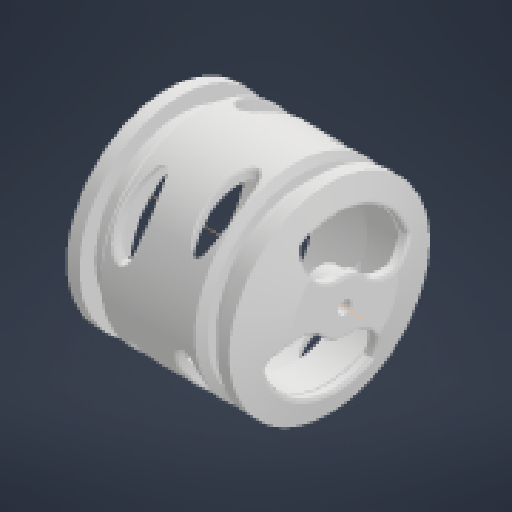
# Autodesk Inventor part: wheel
Saved by Autodesk Inventor 2024 (Build 280153000, 153)
## iProperties
Created: 2023-09-26
Part Number: wheel
Material: Типовые
Document SubType Name: Modeling
Designer: user
Density: 1 g/cm^3
Appearance: По умолчанию
Mass: 47.7551 g
Surface Area: 315.947 cm^2
Volume: 47.7551 cm^3
Author: user
Autodesk Inventor part; units mm, degrees
ref_plane "YZ Plane" through (0, 0, 0) normal (1, 0, 0) x (0, 1, 0)
ref_plane "XZ Plane" through (0, 0, 0) normal (0, 1, 0) x (-1, 0, 0)
sketch "Эскиз1" plane through (0, 0, 0) normal (0, 0, 1) x (1, 0, 0)
  line L0 (0, 0) -> (0, 32)
  line L1 (0, 32) -> (4, 32)
  line L2 (4, 32) -> (4, 27)
  line L3 (4, 27) -> (9, 27)
  line L4 (9, 27) -> (9, 32)
  line L5 (9, 32) -> (43, 32)
  line L6 (43, 32) -> (43, 27)
  line L7 (43, 27) -> (48, 27)
  line L8 (48, 27) -> (48, 32)
  line L9 (48, 32) -> (52, 32)
  line L10 (52, 32) -> (52, 0)
  line L11 (52, 0) -> (0, 0)
  dimension "d0" = 32
  dimension "d1" = 27
  dimension "d2" = 5
  dimension "d3" = 34
  dimension "d4" = 4
  constraints: 24 end point, 8 perpendicular, 6 point on line, 2 collinear, 1 vertical
  measures "d0" distance of L0.start L0.end
  measures "d1" vertical distance of L0.start L2.end
  measures "d2" distance of L2.end L3.end
  measures "d3" distance of L4.end L5.end
  measures "d4" distance of L0.end L1.end
revolve "Вращение1" add sketch "Эскиз1" angle 360 about axis through (52, 0, 0) along (-1, 0, 0)
sketch "Эскиз2" plane through (0, 0, 0) normal (0, 0, 1) x (1, 0, 0)
  line L0 (52, 32) -> (52, -32) projected
  line L1 (52, 32) -> (57, 17)
  line L2 (52, 0) -> (57, 0)
  line L3 (57, 0) -> (57, 17)
  point P0 (0, 0)
  dimension "d6" = 17
  dimension "d7" = 5
  constraints: 6 end point, 1 horizontal, 1 midpoint, 1 perpendicular
  measures "d6" distance of L2.end L1.end
  measures "d7" distance of L2.start L2.end
revolve "Вращение2" add sketch "Эскиз2" angle 360 about axis through (52, 0, 0) along (1, 0, 0)
shell "Оболочка1" thickness 3 removed faces 1 at (0, 9.4449, -4.957)
sketch "Эскиз3" plane through (54, 0, 0) normal (-1, 0, 0) x (0, 0, 1)
  circle A0 centre (0, 0) radius 7.5
  line L0 (-2, -3.4641) -> (-4, 0)
  line L1 (-4, 0) -> (-2, 3.4641)
  line L2 (-2, 3.4641) -> (2, 3.4641)
  line L3 (2, 3.4641) -> (4, 0)
  line L4 (4, 0) -> (2, -3.4641)
  line L5 (2, -3.4641) -> (-2, -3.4641)
  dimension "d10" = 15
  dimension "d11" = 8
  constraints: 12 end point, 2 coincident, 1 centre point, 1 horizontal, 13 other
  measures "d10" diameter of A0
  measures "d11" distance of L0.end L3.end
extrude "Выдавливание1" add sketch "Эскиз3" along normal blind 5.25
sketch "Эскиз4" plane through (54, -3.4641, -2) normal (-1, 0, 0) x (0, 0, 1)
  circle A0 centre (2, 3.4641) radius 7.5 projected
  circle A1 centre (2, 3.4641) radius 2
  dimension "d14" = 4
  constraints: 1 centre point, 1 coincident
  measures "d14" diameter of A1
extrude "Выдавливание2" cut sketch "Эскиз4" against normal through all contours A1
sketch "Эскиз6" plane through (57, 0, 0) normal (1, 0, 0) x (0, 0, -1)
  circle A0 centre (0, 0) radius 24 projected
  arc A1 (5.4637, -6.5114) -> (8.4595, 0.8288) centre (0, 0) ccw
  arc A2 (21.1003, 11.4357) -> (8.4595, 0.8288) centre (18.4118, 1.8039) ccw
  arc A3 (5.4637, -6.5114) -> (7.0727, -22.9342) centre (11.8916, -14.1718) ccw
  line L0 (8.4595, 0.8288) -> (6.271, 23.1662) construction
  line L1 (8.4595, 0.8288) -> (21.1003, 11.4357) construction
  line L2 (5.4637, -6.5114) -> (-11.7297, -20.9383) construction
  line L3 (5.4637, -6.5114) -> (7.0727, -22.9342) construction
  line L4 (0, 0) -> (0, -11.096) construction
  point P0 (0, 0)
  dimension "d26" = 17
  dimension "d29" = 10
  dimension "d31" = 50
  constraints: 10 end point, 10 point on circle, 4 tangent, 3 centre point, 1 coincident, 1 equal radius, 1 parallel, 1 point on line, 1 vertical
  measures "d26" diameter of A1
  measures "d29" radius of A2
  measures "d31" angle of L4 L2
extrude "Выдавливание3" cut sketch "Эскиз6" against normal blind 10 contours A0 A3 A1 A2 picked at (14.0191, -12.4187)
pattern_circular "Круговой массив1" count 2 over 360 about axis through (54.5, 0, 0) along (1, 0, 0) of "Выдавливание3"
ref_plane "РабПлоскость1" through (26, 0, -32) normal (0, 0, 1) x (1, 0, 0)
sketch "Эскиз7" plane through (26, 0, -32) normal (0, 0, 1) x (1, 0, 0)
  ellipse E0 centre (-10, -17) end of major axis (-10, -7) minor radius 4
  ellipse E1 centre (10, 17) end of major axis (10, 7) minor radius 4
  line L0 (-17, 32) -> (-17, -32) construction
  line L1 (17, -32) -> (-17, -32) construction
  line L2 (17, 32) -> (-17, 32) construction
  line L3 (17, 32) -> (17, -32) construction
  point P0 (-26, 0)
  dimension "d41" = 10
  dimension "d42" = 4
  dimension "d37" = 15
  dimension "d38" = 7
  dimension "d39" = 15
  dimension "d40" = 7
  dimension "d43" = 10
  dimension "d44" = 4
  constraints: 1 centre point, 3 other
  measures "d37" distance from line of L1 point (-10, -17)
  measures "d38" distance from line of L0 point (-10, -17)
  measures "d39" distance from line of L2 E1.centre
  measures "d40" distance from line of L3 E1.centre
extrude "Выдавливание4" cut sketch "Эскиз7" along normal up to surface
pattern_circular "Круговой массив2" count 4 over 360 about axis through (26, 0, 0) along (-1, 0, 0) of "Выдавливание4"
chamfer "Фаска1" distance 2 angle 45 2 edges at (9, -32, 0) (43, -32, 0)
chamfer "Фаска2" distance 0.5 angle 45 8 edges at (35.9933, 17.1756, 27) (16.0067, 27, 17.1756) (16.0067, 17.1756, -27) (35.9933, 27, -17.1756) (35.9933, -17.1756, -27) (16.0067, -27, -17.1756) (35.9933, -27, 17.1756) (16.0067, -17.1756, 27)
fillet "Сопряжение1" radius 1 12 edges at (57, -3.2119, -7.8698) (57, 6.3703, -9.5153) (57, -11.2091, -2.3406) (55.7877, -20.2545, -3.9542) (54.6667, -9.069, -22.2206) (55.7877, 11.7034, -16.9974) (57, 3.2119, 7.8698) (57, -6.3703, 9.5153) (57, 11.2091, 2.3406) (55.7877, -11.7034, 16.9974) (55.7877, 20.2545, 3.9542) (54.6667, 9.069, 22.2206)
